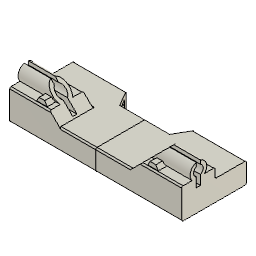
line-follower-mount (Autodesk Fusion 360 design; units mm, degrees)
Autodesk Fusion 360 part; units mm, degrees
note: some values were not read from the file. Set by a fixed rule: which sketch regions a step uses.
sketch "Sketch2" plane through (0, 0, 0) normal (1, 0, 0) x (0, 1, 0)
  line L0 (0, 0) -> (-11.65, 0)
  line L1 (-11.65, 0) -> (-11.65, -7.5)
  line L2 (-11.65, -7.5) -> (-10.25, -7.5)
  line L3 (-9.25, -6.5) -> (-10.05, -6.5)
  line L4 (-10.05, -6.5) -> (-10.05, -4.8)
  line L5 (-10.05, -4.8) -> (-8.45, -4.8)
  line L6 (-8.45, -4.8) -> (-8.45, -3.2)
  line L7 (-8.45, -3.2) -> (-10.05, -3.2)
  line L8 (-10.05, -3.2) -> (-10.05, -1.6)
  line L9 (-10.05, -1.6) -> (0, -1.6)
  line L10 (0, -1.6) -> (0, 0)
  line L11 (-9.25, -6.5) -> (-9.25, -6.7)
  line L12 (-9.25, -6.7) -> (-10.25, -7.5)
  circle A0 centre (-5.65, 5.5) radius 3
  line L13 (9.25, -6.5) -> (10.05, -6.5)
  line L14 (10.05, -1.6) -> (0, -1.6)
  line L15 (10.05, -3.2) -> (10.05, -1.6)
  line L16 (0, -1.6) -> (0, 0)
  line L17 (8.45, -3.2) -> (10.05, -3.2)
  line L18 (9.25, -6.5) -> (9.25, -6.7)
  line L19 (0, 0) -> (11.65, 0)
  line L20 (10.05, -4.8) -> (8.45, -4.8)
  line L21 (9.25, -6.7) -> (10.25, -7.5)
  line L22 (8.45, -4.8) -> (8.45, -3.2)
  line L23 (10.05, -6.5) -> (10.05, -4.8)
  line L24 (11.65, -7.5) -> (10.25, -7.5)
  line L25 (11.65, 0) -> (11.65, -7.5)
  circle A1 centre (-5.65, 5.5) radius 1.75
  line L26 (-11.65, 3.5) -> (0.35, 3.5)
  line L27 (0.35, 3.5) -> (0.35, 0)
  line L28 (0.35, 0) -> (-11.65, 0)
  line L29 (-11.65, 0) -> (-11.65, 3.5)
  line L30 (-6.4, 9.5) -> (-4.9, 9.5)
  line L31 (-4.9, 9.5) -> (-4.9, 0.5)
  line L32 (-4.9, 0.5) -> (-6.4, 0.5)
  line L33 (-6.4, 0.5) -> (-6.4, 9.5)
  line L34 (-11.65, -7.5) -> (11.65, -7.5)
  point P0 (-5.65, 0.5)
  point P1 (-5.65, 3.5)
  dimension "d3" = 1.6
  dimension "d5" = 0.2
  dimension "d6" = 1.4
  dimension "d7" = 1
  dimension "d8" = 0.8
  dimension "d9" = 7.5
  dimension "d10" = 10.05
  dimension "d11" = 1.6
  dimension "d12" = 1.6
  dimension "d13" = 1.6
  dimension "d14" = 1.7
  dimension "d15" = 0.8
  dimension "d17" = 5.5
  dimension "d18" = 3.5
  dimension "d19" = 2
  dimension "d20" = 12
  dimension "d21" = 5
  dimension "d22" = 1.5
  dimension "d23" = 9
  constraint coincident L0.start L10.end
  constraint horizontal L0
  constraint perpendicular L0 L1
  constraint perpendicular L1 L2
  constraint parallel L2 L3
  constraint perpendicular L3 L4
  constraint perpendicular L4 L5
  constraint perpendicular L3 L6
  constraint perpendicular L4 L7
  constraint perpendicular L7 L8
  constraint perpendicular L4 L9
  constraint perpendicular L0 L10
  constraint perpendicular L3 L11
  constraint collinear L4 L8
  constraint symmetric L0.start L10 L16.end
  constraint symmetric L0.end L10 L19.end
  constraint symmetric L1.end L10 L24.start
  constraint symmetric L2.end L10 L21.end
  constraint symmetric L3.start L10 L13.start
  constraint symmetric L3.end L10 L13.end
  constraint symmetric L4.end L10 L20.start
  constraint symmetric L5.end L10 L20.end
  constraint symmetric L6.end L10 L17.start
  constraint symmetric L7.end L10 L15.start
  constraint symmetric L8.end L10 L14.start
  constraint symmetric L9.end L10 L14.end
  constraint symmetric L10 L11.end L18.end
  constraint concentric A0 A1
  constraint horizontal L26
  constraint vertical L27
  constraint horizontal L28
  constraint vertical L29
  constraint coincident L19 L27.end
  constraint horizontal L30
  constraint vertical L31
  constraint horizontal L32
  constraint vertical L33
  constraint midpoint L32 P0
  constraint vertical A0.centre P0
  constraint midpoint L26 P1
  constraint vertical A0.centre P1
  constraint coincident L0.end L1.start
  measures "d3" distance of L9.end L0.start
  measures "d5" distance of L3.start L11.end
  measures "d6" distance of L1.end L2.end
  measures "d7" horizontal distance of L2.end L11.end
  measures "d8" vertical distance of L2.end L11.end
  measures "d9" distance of L0.end L1.end
  measures "d10" distance of L8.end L9.end
  measures "d11" distance of L7.end L8.end
  measures "d12" distance of L6.end L7.end
  measures "d13" distance of L5.end L6.end
  measures "d14" distance of L3.end L4.end
  measures "d15" distance of L3.start L3.end
  measures "d17" vertical distance of L0.start A0.centre
  measures "d18" diameter of A1
  measures "d19" vertical distance of A0.centre L26.end
  measures "d20" distance of L26.start L26.end
  measures "d21" vertical distance of A0.centre L32.end
  measures "d22" distance of L30.start L30.end
  measures "d23" distance of L30.end L31.end
  measures "d74" distance of L0.start
  measures "d75" distance of L0.start
  measures "d79" distance of L0.start
extrude "Extrude1" add sketch "Sketch2" along normal blind 31 contours L0 L1 L2 L3 L4 L5 L6 L7 L8 L9 L10 L11 L12 L16 L28 L34 | L10 L13 L14 L15 L16 L17 L18 L19 L20 L21 L22 L23 L24 L25 L28 L34 | L0 A0 L19 L26 L27 L28 L29 L31 L32 L33 | A0 L26 L33 | A0 A1 L26 L33 | A0 A1 L26 L31 | A0 L26 L31 makes body 1
extrude "Extrude4" add sketch "Sketch2" along normal blind 1 from surface at 30 contours L0 L1 L2 L3 L4 L5 L6 L7 L8 L9 L10 L11 L12 L16 L28 L34 | L10 L13 L14 L15 L16 L17 L18 L19 L20 L21 L22 L23 L24 L25 L28 L34 | L3 L4 L5 L6 L7 L8 L9 L11 L12 L13 L14 L15 L17 L18 L20 L21 L22 L23 L34 bodies 1
sketch "Sketch3" plane through (0, 0, 0) normal (0, 1, 0) x (1, 0, 0)
  line L0 (0, 0) -> (13, 0)
  line L1 (13, 0) -> (22, -9)
  line L2 (22, -9) -> (0, -9)
  line L3 (0, -9) -> (0, 0)
  line L4 (18.966, -5) -> (21.034, -5)
  line L5 (21.034, -5) -> (21.9, -3.5)
  line L6 (21.9, -3.5) -> (18.1, -3.5)
  line L7 (18.1, -3.5) -> (18.966, -5)
  point P0 (0, -9)
  point P1 (20, -3.5)
  dimension "d28" = 135
  dimension "d37" = 9
  dimension "d38" = 22
  dimension "d70" = 120
  dimension "d71" = 120
  dimension "d72" = 1.5
  dimension "d73" = 3.8
  dimension "d74" = 20
  dimension "d75" = 3.5
  constraint coincident L0.start L3.end
  constraint horizontal L0
  constraint vertical L0.start L2.end
  constraint coincident P0 L2.end
  constraint horizontal L2
  constraint horizontal L4
  constraint parallel L4 L6
  constraint midpoint L6 P1
  measures "d28" angle of L0 L1
  measures "d37" distance of P0 L0.start
  measures "d38" distance of L1.end P0
  measures "d70" angle of L4 L5
  measures "d71" angle of L4 L7
  measures "d72" distance of L4 L6
  measures "d73" distance of L5.end L6.end
  measures "d74" horizontal distance of L0.start P1
  measures "d75" vertical distance of L0.start P1
extrude "Extrude2" cut sketch "Sketch3" along normal through all and the other way through all contours L0 L1 L2 L3 bodies 1
sketch "Sketch4" plane through (0, 0, 0) normal (0, 0, 1) x (-1, 0, 0)
  line L0 (0, 11.65) -> (-13, 11.65)
  line L1 (-13, 11.65) -> (-13, -0.35)
  line L2 (-13, -0.35) -> (-31, -0.35)
  line L3 (-31, -0.35) -> (-31, -11.65)
  line L4 (-31, -11.65) -> (0, -11.65)
  line L5 (0, -11.65) -> (0, 11.65)
  line L6 (-11.3383, -10.05) -> (-13.9363, -8.55)
  line L7 (-13.9363, -8.55) -> (-13.9363, -6)
  line L8 (-13.9363, -6) -> (-9, -6)
  line L9 (0, -12) -> (0, 0)
  line L10 (0, -6) -> (-9, -6)
  line L11 (-9, -6) -> (-12.4641, -12)
  line L12 (-9, -6) -> (-1.7604, -6) construction
  line L13 (-12.4641, -12) -> (0, -12)
  dimension "d59" = 1.6
  dimension "d60" = 3
  dimension "d68" = 12
  dimension "d79" = 6
  dimension "d81" = 9
  dimension "d82" = 120
  constraint perpendicular L4 L7
  constraint horizontal L8
  constraint coincident L9.end origin
  constraint coincident L5 L10.start
  constraint coincident L9 L10.start
  constraint perpendicular L9 L10
  constraint horizontal L12
  constraint horizontal L13
  constraint coincident L6.start L11
  constraint coincident L8.end L11
  constraint perpendicular L6 L11
  constraint collinear L8 L10
  measures "d59" vertical distance of L3.end L6.start
  measures "d60" distance of L6.start L6.end
  measures "d68" distance of L9.start L9.end
  measures "d79" distance of L9.end L10.start
  measures "d81" distance of L10.start L8.end
  measures "d82" angle of L11 L12
extrude "Extrude3" cut sketch "Sketch4" against normal blind 25 contours L4 L5 L9 L10 L11 bodies 1
extrude "Extrude6" cut sketch "Sketch4" against normal blind 11.5 from surface at -2 contours L6 L7 L8 L11 bodies 1
fillet "Fillet1" radius 0.5 7 edges at (23.75, -11.65, 3.5) (23.75, 0.35, 3.5) (21.631, 11.65, 0) (22, 0.35, 0) (21.631, 11.65, -7.5) (15.5, -11.65, -7.5) (6.5, -11.65, 0) on bodies 1
extrude "Extrude7" add sketch "Sketch3" against normal blind 3 from surface at -8 contours L4 L5 L6 L7 bodies 1
mirror "Mirror1" about plane through (0, 0, 0) normal (1, 0, 0) of bodies 1 makes body 2
